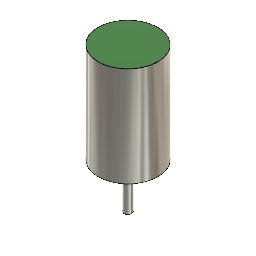
motor v1 (Autodesk Fusion 360 design; units mm, degrees)
Autodesk Fusion 360 part; units mm, degrees
sketch "スケッチ1" plane through (0, 0, 0) normal (0, 0, 1) x (1, 0, 0)
  circle A0 centre (0, 0) radius 3
  circle A1 centre (0, 0) radius 0.4
  dimension "d1" = 6
  dimension "d7" = 0.8
  measures "d1" diameter of A0
  measures "d7" diameter of A1
extrude "押し出し1" add sketch "スケッチ1" along normal blind 10 contours A0 | A1 makes body 1
extrude "押し出し1'" add sketch "スケッチ1" against normal blind 4.5 separate body contours A1 makes body 2 in component "Component'"
component "Component'" placed x (1, 0, 0) y (0, 1, 0) z (0, 0, 1) at (0, 0, 0)
